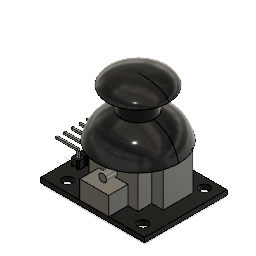
joystickModule (Autodesk Fusion 360 design; units mm, degrees)
Autodesk Fusion 360 part; units mm, degrees
note: some values were not read from the file. Chosen so that the rebuilt part matches the saved one: which face or edge a step refers to. Set by a fixed rule: which sketch regions a step uses; the direction of a hole.
sketch "PCB" plane through (0, 0, 0) normal (0, 1, 0) x (1, 0, 0) in component "PCB"
  line L0 (0, 0) -> (34, 0)
  line L1 (34, 0) -> (34, -27)
  line L2 (34, -27) -> (0, -27)
  line L3 (0, -27) -> (0, 0)
  line L4 (0, -7.5) -> (3, -7.5) construction
  line L5 (3, 0) -> (3, -7.5) construction
  line L6 (3, -7.5) -> (3, -10.04) construction
  line L7 (3, -10.04) -> (3, -12.58) construction
  line L8 (3, -12.58) -> (3, -15.12) construction
  line L9 (3, -15.12) -> (3, -17.66) construction
  line L10 (34, -3.3375) -> (29.825, -3.3375) construction
  line L11 (29.825, -3.3375) -> (29.825, 0) construction
  line L12 (29.825, -27) -> (29.825, -23.4125) construction
  line L13 (0, -23.4125) -> (5.2875, -23.4125) construction
  dimension "d1" = 34
  dimension "d2" = 27
  dimension "d3" = 3
  dimension "d4" = 7.5
  dimension "d5" = 2.54
  dimension "d6" = 2.54
  dimension "d7" = 2.54
  dimension "d8" = 2.54
  dimension "d9" = 4.175
  dimension "d10" = 3.3375
  dimension "d11" = 3.5875
  dimension "d12" = 5.2875
  dimension "d100" = 0
  dimension "d101" = 0
  dimension "d102" = 0
  dimension "d103" = 0
  measures "d10" distance of L0.start
  measures "d12" distance of L0.start
extrude "Extrude1" add sketch "PCB" along normal blind 1.6 makes body 1 in component "PCB"
hole "Hole1" at (5.2875, 0, 3.3375) at (5.2875, 0, 23.4125) at (29.825, 0, 3.3375) at (29.825, 0, 23.4125) direction (0, 1, 0) diameter 3.175 depth 1.6 tip angle 118 bodies 1 in component "PCB"
hole "Hole2" at (3, 0, 17.66) at (3, 0, 15.12) at (3, 0, 12.58) at (3, 0, 10.04) at (3, 0, 7.5) direction (0, 1, 0) diameter 1 depth 1.6 tip angle 118 bodies 1 in component "PCB"
sketch "Sketch1" plane through (0, 0, 0) normal (0, 1, 0) x (1, 0, 0) in component "Pin"
  line L0 (0, 0) -> (7.239, 0)
  line L1 (7.239, 0) -> (7.239, -7.62)
  line L2 (0, -0.635) -> (0, 0)
  line L3 (7.239, -7.62) -> (6.604, -7.62)
  line L4 (6.604, -7.62) -> (6.604, -0.635)
  line L5 (0, -0.635) -> (6.604, -0.635)
  dimension "d2_1" = 0.635
  dimension "d3_1" = 7.239
  dimension "d23" = 7.62
  measures "d3_1" distance of L0.start
extrude "Extrude1'" add sketch "Sketch1" along normal blind 0.635 separate body makes body 2 in component "Pin"
chamfer "Chamfer1" distance 0.1905 angle 45 8 edges at (6.9215, 0.635, 7.62) (6.9215, 0, 7.62) (6.604, 0.3175, 7.62) (7.239, 0.3175, 7.62) (0, 0.3175, 0.635) (0, 0.635, 0.3175) (0, 0.3175, 0) (0, 0, 0.3175) on bodies 2 in component "Pin"
sketch "Sketch1 (2)" plane through (0, 0, 0) normal (0, 1, 0) x (1, 0, 0) in component "Plastic"
  line L0 (0, -0.4445) -> (0, -0.1905)
  line L1 (0, -0.3175) -> (2.921, -0.3175) construction
  line L2 (2.921, -1.0795) -> (2.921, 0.4445)
  line L3 (0.1905, 0) -> (7.239, 0) construction
  line L4 (2.921, 0.4445) -> (2.921, 0.9525) construction
  line L5 (2.921, -1.0795) -> (2.921, -1.5875) construction
  line L6 (2.921, 0.4445) -> (2.286, 0.4445)
  line L7 (2.921, -1.0795) -> (2.286, -1.0795)
  line L8 (2.286, -1.0795) -> (2.286, -1.5875)
  line L9 (2.286, 0.4445) -> (2.286, 0.9525)
  line L10 (2.286, 0.9525) -> (4.826, 0.9525)
  line L11 (4.826, 0.9525) -> (4.826, -1.5875)
  line L12 (2.286, -1.5875) -> (4.826, -1.5875)
  dimension "d7_1" = 2.921
  dimension "d8_1" = 1.524
  dimension "d9_1" = 0.508
  dimension "d11_1" = 0.635
  dimension "d12_1" = 2.54
  measures "d7_1" distance of origin
extrude "Extrude1''" add sketch "Sketch1 (2)" along normal mid plane 2.54 from surface at 0.3175 separate body makes body 3 in component "Plastic"
chamfer "Chamfer1'" distance 0.4 angle 45 4 edges at (3.556, 1.5875, -0.9525) (3.556, -0.9525, -0.9525) (3.556, 1.5875, 1.5875) (3.556, -0.9525, 1.5875) on bodies 3 in component "Plastic"
sketch "Sketch1 (3)" plane through (0, 0, 0) normal (0, 0, 1) x (1, 0, 0) in component "Pins bent alt. male v4"
  line L0 (0, 0.1905) -> (0, 0.4445)
  line L1 (0, 0.3175) -> (0, 14)
fillet "Fillet1" radius 0.5 1 edges at (7.239, 0.3175, 0) on bodies 2 in component "Pin"
other "PathPattern1" in component "Header"
sketch "Sketch1 (4)" plane through (0, 1.6, 0) normal (0, 1, 0) x (-1, 0, 0) in component "MainPart"
  circle A0 centre (-3, 10.04) radius 0.5
  circle A1 centre (-3, 15.12) radius 0.5
  circle A2 centre (-3, 17.66) radius 0.5
  circle A3 centre (-3, 12.58) radius 0.5
  circle A4 centre (-3, 7.5) radius 0.5
  circle A5 centre (-29.825, 3.3375) radius 1.5875
  circle A6 centre (-5.2875, 3.3375) radius 1.5875
  circle A7 centre (-5.2875, 23.4125) radius 1.5875
  circle A8 centre (-29.825, 23.4125) radius 1.5875
  line L0 (0, 27) -> (-34, 27)
  line L1 (-34, 27) -> (-34, 0)
  line L2 (-34, 0) -> (0, 0)
  line L3 (0, 0) -> (0, 27)
  line L4 (-25.6, 20.75) -> (-9.6, 20.75)
  line L5 (-9.6, 20.75) -> (-9.6, 4.75)
  line L6 (-19, 4.75) -> (-19, 1.05) construction
  line L7 (-14.15, 1.05) -> (-23.85, 1.05)
  line L8 (-23.85, 1.05) -> (-23.85, 4.75)
  line L9 (-14.15, 1.05) -> (-14.15, 4.75)
  line L10 (-9.6, 4.75) -> (-14.15, 4.75)
  line L11 (-23.85, 4.75) -> (-25.6, 4.75)
  line L12 (-14.15, 4.75) -> (-19, 4.75) construction
  line L13 (-19, 4.75) -> (-23.85, 4.75) construction
  line L14 (-25.6, 11.3996) -> (-29.3, 11.3996) construction
  line L15 (-29.3, 6.5496) -> (-29.3, 16.2496)
  line L16 (-29.3, 16.2496) -> (-25.6, 16.2496)
  line L17 (-29.3, 6.5496) -> (-25.6, 6.5496)
  line L18 (-25.6, 4.75) -> (-25.6, 6.5496)
  line L19 (-25.6, 16.2496) -> (-25.6, 20.75)
  line L20 (-25.6, 6.5496) -> (-25.6, 11.3996) construction
  line L21 (-25.6, 11.3996) -> (-25.6, 16.2496) construction
  line L22 (-17.6, 20.75) -> (-17.6, 27) construction
  line L23 (-12.9, 27) -> (-22.3, 27)
  line L24 (-12.9, 27) -> (-12.9, 20.75)
  line L25 (-22.3, 27) -> (-22.3, 20.75)
  line L26 (-34, 27) -> (0, 27)
  line L27 (-34, 6.5466) -> (-25.6, 6.5466) construction
  dimension "d33" = 16
  dimension "d34" = 16
  dimension "d35" = 3.7
  dimension "d36" = 9.7
  dimension "d37" = 6.25
  dimension "d38" = 8.4
  dimension "d39" = 9.4
  measures "d36" distance of L2.end
  measures "d39" distance of L2.end
extrude "Extrude1'''" add sketch "Sketch1 (4)" along normal blind 12.5 separate body contours L4 L5 L7 L8 L9 L10 L11 L15 L16 L17 L18 L19 makes body 4 in component "MainPart"
extrude "Extrude2" add sketch "Sketch1 (4)" along normal blind 6 contours L0 L4 L23 L24 L25 L26 bodies 4 in component "MainPart"
sketch "Sketch2" plane through (0, 0, 20.75) normal (0, 0, 1) x (1, 0, 0) in component "MainPart"
  line L0 (22.3, 7.6) -> (22.3, 1.6)
  line L1 (22.3, 1.6) -> (25.6, 1.6)
  line L2 (25.6, 1.6) -> (25.6, 14.1)
  line L3 (25.6, 14.1) -> (9.6, 14.1)
  line L4 (9.6, 14.1) -> (9.6, 1.6)
  line L5 (9.6, 1.6) -> (12.9, 1.6)
  line L6 (12.9, 1.6) -> (12.9, 7.6)
  line L7 (12.9, 7.6) -> (22.3, 7.6)
  line L8 (17.6, 7.6) -> (17.6, 8.85) construction
  circle A0 centre (17.6, 8.85) radius 1.25
  dimension "d44" = 1.25
  dimension "d45" = 2.5
  measures "d45" diameter of A0
extrude "Extrude3" add sketch "Sketch2" along normal blind 3.5 separate body contours A0 makes body 5 in component "MainPart"
sketch "Sketch3" plane through (0, 14.1, 0) normal (0, 1, 0) x (-1, 0, 0) in component "MainPart"
  line L0 (-29.3, 6.5496) -> (-25.6, 6.5496)
  line L1 (-25.6, 6.5496) -> (-25.6, 4.75)
  line L2 (-25.6, 4.75) -> (-23.85, 4.75)
  line L3 (-23.85, 4.75) -> (-23.85, 1.05)
  line L4 (-23.85, 1.05) -> (-14.15, 1.05)
  line L5 (-14.15, 1.05) -> (-14.15, 4.75)
  line L6 (-14.15, 4.75) -> (-9.6, 4.75)
  line L7 (-9.6, 4.75) -> (-9.6, 20.75)
  line L8 (-9.6, 20.75) -> (-25.6, 20.75)
  line L9 (-25.6, 20.75) -> (-25.6, 16.2496)
  line L10 (-25.6, 16.2496) -> (-29.3, 16.2496)
  line L11 (-29.3, 16.2496) -> (-29.3, 6.5496)
  line L12 (-9.6, 12.75) -> (-17.6, 12.75) construction
  line L13 (-17.6, 20.75) -> (-17.6, 12.75) construction
hole "Hole1'" at (17.6, 14.1, 12.75) direction (0, -1, 0) diameter 7.5 depth 5.25 tip angle 180 bodies 4 in component "MainPart"
sketch "Sketch1 (5)" plane through (0, 8.85, 0) normal (0, 1, 0) x (-1, 0, 0) in component "Stick"
  circle A0 centre (-17.6, 12.75) radius 3.75
  line L0 (-17, 12.75) -> (-18.2, 12.75) construction
  line L1 (-18.2, 11.8) -> (-17, 11.8)
  line L2 (-17, 11.8) -> (-17, 13.7)
  line L3 (-17, 13.7) -> (-18.2, 13.7)
  line L4 (-18.2, 13.7) -> (-18.2, 11.8)
  dimension "d52" = 1.2
  dimension "d53" = 1.9
extrude "Extrude1''''" add sketch "Sketch1 (5)" along normal blind 12.45 separate body contours L1 L2 L3 L4 makes body 6 in component "Stick"
sketch "Sketch1 (6)" plane through (0, 0, 0) normal (0, 0, 1) x (1, 0, 0) in component "Knob"
  line L0 (0, 0) -> (0, 2.5) construction
  line L1 (5.25, 2.5) -> (5.25, -2.5)
  line L2 (0, 0) -> (5.25, 0) construction
  line L3 (5.25, -2.5) -> (5.25, -11) construction
  line L4 (0, -11) -> (13.25, -11) construction
  spline S0 degree 2 poles (5.25, -2.5) (11.638, -4.7439) (13.25, -11) knots 0 0 0 1.219775 1.219775 1.219775 weights 1 1.317188 1
  line L5 (0, 2.5) -> (0, 3)
  line L6 (0, 3) -> (0, 4.5) construction
  line L7 (0, 4.5) -> (10, 4.5) construction
  line L8 (5.25, 2.5) -> (10, 4.5)
  line L9 (0, 4.5) -> (0, 8) construction
  spline S1 degree 2 poles (0, 8) (9.4466, 8) (10, 4.5) knots 0 0 0 1.100734 1.100734 1.100734 weights 1 0.839133 1
  line L10 (0, -11) -> (0, -7.5) construction
  line L11 (0, -7.5) -> (3, -7.5)
  line L12 (3, -7.5) -> (5.0689, -3.4835)
  line L13 (0, -7.5) -> (0, 8)
  spline S2 degree 3 poles (4.9186, -3.4435) (6.7304, -4.0799) (7.8476, -4.6631) (8.7321, -5.2976) (9.732, -6.0149) (10.4112, -6.775) (11.0183, -7.8716) (11.4807, -8.7068) (11.89, -9.7297) (12.2816, -11.2495) knots 0 0 0 0 0.407745 0.407745 0.407745 0.868685 0.868685 0.868685 1.219775 1.219775 1.219775 1.219775
  line L14 (13.25, -11) -> (12.216, -11)
  dimension "d66" = 5.25
  dimension "d67" = 5
  dimension "d68" = 8.5
  dimension "d69" = 13.25
  dimension "d70" = 1.5
  dimension "d71" = 10
  dimension "d72" = 3.5
  dimension "d74" = 3.5
  dimension "d75" = 3
  dimension "d117" = 1
  measures "d66" distance of L0.start
  measures "d117" distance of S0
revolve "Revolve1" add sketch "Sketch1 (6)" angle 360 about axis through (0, -7.5, 0) along (0, 1, 0) separate body makes body 7 in component "Knob"
sketch "Sketch2 (2)" plane through (0, -7.5, 0) normal (0, -1, 0) x (1, 0, 0) in component "Knob"
  circle A0 centre (0, 0) radius 3
  line L0 (-0.6, 0) -> (0.6, 0) construction
  line L1 (0.6, 0.95) -> (-0.6, 0.95)
  line L2 (-0.6, 0.95) -> (-0.6, -0.95)
  line L3 (-0.6, -0.95) -> (0.6, -0.95)
  line L4 (0.6, -0.95) -> (0.6, 0.95)
  dimension "d77" = 1.2
  dimension "d78" = 1.9
extrude "Extrude1'''''" cut sketch "Sketch2 (2)" against normal blind 4 contours L1 L2 L3 L4 bodies 7 in component "Knob"
component "Joystick" placed x (1, 0, 0) y (0, 1, 0) z (0, 0, 1) at (0, 0, 0)
component "PCB" placed x (1, 0, 0) y (0, 1, 0) z (0, 0, 1) at (0, 0, 0) in component "Joystick"
component "Pins bent alt. male v4" placed x (0, 1, 0) y (0, 0, -1) z (-1, 0, 0) at (-5, 0, 18) in component "Joystick"
component "MainPart" placed x (1, 0, 0) y (0, 1, 0) z (0, 0, 1) at (0, 0, 0) in component "Joystick"
component "Knob" placed x (1, 0, 0) y (0, 1, 0) z (0, 0, 1) at (17.6, 24.8, 12.75) in component "Joystick"
component "Stick" placed x (1, 0, 0) y (0, 1, 0) z (0, 0, 1) at (0, 0, 0) in component "MainPart"
component "Header" placed x (1, 0, 0) y (0, 1, 0) z (0, 0, 1) at (-0.686, 0.0225, -8.3175) in component "Pins bent alt. male v4"
component "Header" placed x (1, 0, 0) y (0, 1, 0) z (0, 0, 1) at (-0.686, 2.5625, -8.3175) in component "Pins bent alt. male v4"
component "Header" placed x (1, 0, 0) y (0, 1, 0) z (0, 0, 1) at (-0.686, 5.1025, -8.3175) in component "Pins bent alt. male v4"
component "Header" placed x (1, 0, 0) y (0, 1, 0) z (0, 0, 1) at (-0.686, 7.6425, -8.3175) in component "Pins bent alt. male v4"
component "Header" placed x (1, 0, 0) y (0, 1, 0) z (0, 0, 1) at (-0.686, 10.1825, -8.3175) in component "Pins bent alt. male v4"
component "Pin" placed x (1, 0, 0) y (0, 1, 0) z (0, 0, 1) at (0, 0, 0) in component "Header"
component "Plastic" placed x (1, 0, 0) y (0, 1, 0) z (0, 0, 1) at (0, 0, 0) in component "Header"
equation "d9 = 1 mm + 0.125 in"
equation "d10 = 1.75 mm + ( 0.125 in / 2 )"
equation "d11 = 2 mm + ( 0.125 in / 2 )"
equation "d12 = 3.7 mm + ( 0.125 in / 2 )"
equation "d44 = ( 2.5 / 2 ) * 1 mm"
equation "d54 = 5.25 mm + 7.2 mm"
equation "d66 = ( 10.5 / 2 ) * 1 mm"
equation "d69 = 26.5 mm / 2"
equation "d71 = ( 20 / 2 ) * 1 mm"
equation "d72 = 18.5 mm - 1.5 mm - 5 mm - 8.5 mm"
equation "pinCount = 5"
equation "d13_1 = 0.025 in / 2"
equation "d19_1 = pinCount"
equation "d21 = pinCount"
